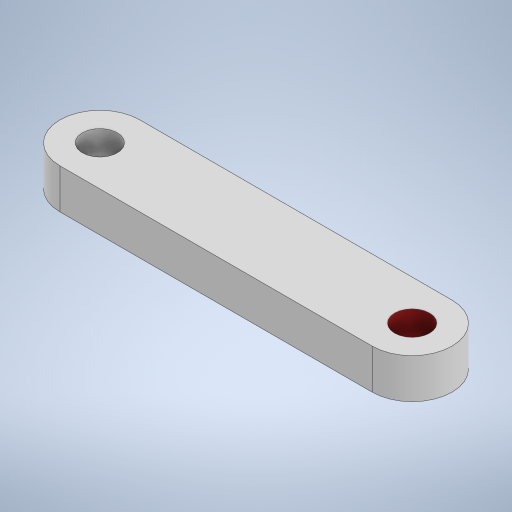
# Autodesk Inventor part: mechanism_1
Saved by Autodesk Inventor 2023 (Build 270158000, 158)
## iProperties
Created: 2024-07-18
Part Number: mechanism_1
Material: Generic
Document SubType Name: Modeling
Designer: Swoby
Density: 1 g/cm^3
Appearance: Default
Author: Swoby
Autodesk Inventor part; units mm, degrees
ref_plane "YZ Plane" through (0, 0, 0) normal (1, 0, 0) x (0, 1, 0)
ref_plane "XZ Plane" through (0, 0, 0) normal (0, 1, 0) x (-1, 0, 0)
ref_plane "XY Plane" through (0, 0, 0) normal (0, 0, 1) x (1, 0, 0)
sketch "Sketch1" plane through (0, 0, 0) normal (0, 1, 0) x (-1, 0, 0)
  circle A0 centre (0, 0) radius 1.75
  circle A1 centre (-31.322, 0) radius 1.75
  line L0 (0, 0) -> (-31.322, 0)
  line L1 (4, 0) -> (-35.322, 0) construction
  line L2 (0, -4) -> (-31.322, -4)
  line L3 (-31.322, 4) -> (0, 4)
  arc A2 (0, -4) -> (0, 4) centre (0, 0) ccw
  arc A3 (-31.322, 4) -> (-31.322, -4) centre (-31.322, 0) ccw
  point P0 (-15.661, 0)
  dimension "d0" = 31.322
  dimension "d1" = 3.5
  dimension "d2" = 3.5
  dimension "d3" = 4
  constraints: 10 end point, 6 point on circle, 4 centre point, 4 tangent, 3 coincident, 2 horizontal, 2 point on line, 1 midpoint, 1 parallel
  measures "d0" distance of L0.end point (0, 0)
  measures "d1" diameter of A0
  measures "d2" diameter of A1
  measures "d3" radius of A2
extrude "Extrusion1" add sketch "Sketch1" along normal blind 4
body "Solid1"
